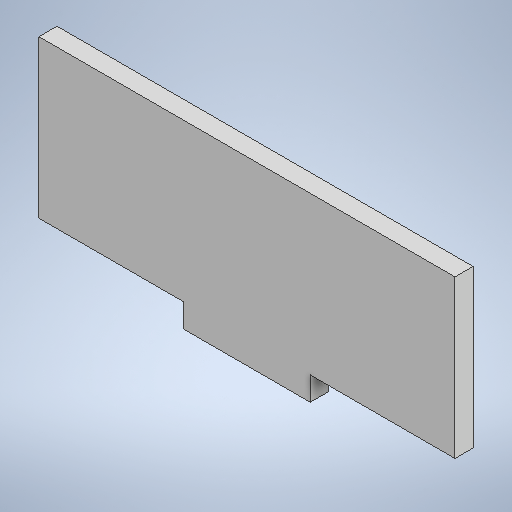
# Autodesk Inventor part: front
Saved by Autodesk Inventor 2025.3 (Build 293356030, 356C)
## iProperties
Created: 2026-06-25
Part Number: front
Material: Generic
Document SubType Name: Modeling
Designer: user
Density: 1 g/cm^3
Appearance: Default
Author: user
Autodesk Inventor part; units mm, degrees
ref_plane "YZ Plane" through (0, 0, 0) normal (1, 0, 0) x (0, 1, 0)
ref_plane "XZ Plane" through (0, 0, 0) normal (0, 1, 0) x (-1, 0, 0)
ref_plane "XY Plane" through (0, 0, 0) normal (0, 0, 1) x (1, 0, 0)
sketch "Sketch1" plane through (0, 0, 0) normal (0, 0, 1) x (1, 0, 0)
  line L0 (80, 0) -> (150, 0)
  line L1 (230, 0) -> (230, 100)
  line L2 (230, 100) -> (0, 100)
  line L3 (0, 100) -> (0, 13.0816)
  line L4 (80, 0) -> (150, 0)
  line L5 (150, 0) -> (150, 13.0816)
  line L6 (80, 13.0816) -> (80, 0)
  line L7 (80, 13.0816) -> (0, 13.0816)
  line L8 (150, 13.0816) -> (230, 13.0816)
  point P0 (0, 0)
  dimension "d2" = 230
  dimension "d3" = 100
  constraints: 18 end point, 3 parallel, 3 perpendicular, 2 horizontal, 1 point on line
  measures "d2" distance of L2.end L1.end
  measures "d3" distance of L1.end L1.start
extrude "Extrusion1" add sketch "Sketch1" along normal blind 10
body "Solid1"
